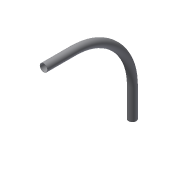
# Autodesk Inventor part: sweep
Saved by Autodesk Inventor 2016 (Build 200138000, 138)
## iProperties
Created: 2014-03-12
Part Number: sweep
Material: Generic
Document SubType Name: Modeling
Designer: Dave
Density: 1 g/cm^3
Appearance: Default
Author: Dave
Autodesk Inventor part; units mm, degrees
ref_plane "YZ Plane" through (0, 0, 0) normal (1, 0, 0) x (0, 1, 0)
ref_plane "XZ Plane" through (0, 0, 0) normal (0, 1, 0) x (-1, 0, 0)
ref_plane "XY Plane" through (0, 0, 0) normal (0, 0, 1) x (1, 0, 0)
sketch "Sketch1" plane through (0, 0, 0) normal (0, 1, 0) x (-1, 0, 0)
  circle A0 centre (0, 0) radius 20
  circle A1 centre (0, 0) radius 18.5
  dimension "d0" = 40
  dimension "d1" = 1.5
  constraints: 2 centre point, 1 coincident
  measures "d0" diameter of A0
  measures "d1" radial gap between concentric circles of A1 A0
extrude "Extrusion1" add sketch "Sketch1" along normal blind 152.4
sketch "Sketch4" plane through (0, 152.4, 0) normal (0, 1, 0) x (1, 0, 0)
  circle A0 centre (0, 0) radius 18.5 projected
  circle A1 centre (0, 0) radius 20 projected
  point P0 (-20, 0)
  constraints: 1 horizontal alignment, 1 other
ref_plane "Work Plane4" through (-20, 152.4, 0) normal (-1, 0, 0) x (0, -1, 0)
sketch "Sketch8" plane through (-20, 152.4, 0) normal (-1, 0, 0) x (0, -1, 0)
  line L0 (0, 0) -> (0, 304.8) construction
  arc A0 (-304.8, 304.8) -> (0, 0) centre (0, 304.8) ccw
  line L1 (0, 304.8) -> (-304.8, 304.8) construction
  point P0 (152.4, 0)
  dimension "d7" = 304.8
  constraints: 4 end point, 2 point on circle, 1 centre point, 1 coincident, 1 perpendicular, 1 vertical
  measures "d7" distance of L0.start L0.end
sweep "Sweep1" add profiles "Sketch4" path "Sketch8"
sketch "Sketch9" plane through (0, 457.2, 304.8) normal (0, 0, 1) x (1, 0, 0)
  circle A0 centre (0, 0) radius 18.5 projected
  circle A1 centre (0, 0) radius 20 projected
  point P0 (0, -457.2)
extrude "Extrusion2" add sketch "Sketch9" along normal blind 152.4
body "Solid1"
